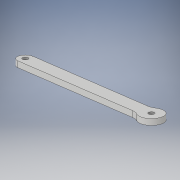
# Autodesk Inventor part: 連接1
Saved by Autodesk Inventor 2017 (Build 210142000, 142)
## iProperties
Part Number: 連接1
Material: 一般
Document SubType Name: Modeling
Designer: User
Density: 1 g/cm^3
Appearance: 預設
Author: User
Autodesk Inventor part; units mm, degrees
ref_plane "YZ Plane" through (0, 0, 0) normal (1, 0, 0) x (0, 1, 0)
ref_plane "XZ Plane" through (0, 0, 0) normal (0, 1, 0) x (-1, 0, 0)
ref_plane "XY Plane" through (0, 0, 0) normal (0, 0, 1) x (1, 0, 0)
sketch "草圖1" plane through (0, 0, 0) normal (0, 1, 0) x (-1, 0, 0)
  circle A0 centre (0, 0) radius 1.5
  circle A1 centre (0, 0) radius 4
  line L0 (0, 0) -> (-80, 0)
  circle A2 centre (-80, 0) radius 1.5
  arc A3 (-76.9095, 5.1429) -> (-76.9095, -5.1429) centre (-80, 0) ccw
  line L1 (0, 4) -> (-72.7889, 4)
  line L2 (0, -4) -> (-72.7889, -4)
  arc A4 (-76.9095, 5.1429) -> (-72.7889, 4) centre (-72.7889, 12) ccw
  arc A5 (-72.7889, -4) -> (-76.9095, -5.1429) centre (-72.7889, -12) ccw
  point P0 (-75.5279, 4)
  point P1 (-75.5279, -4)
  dimension "d0" = 3
  dimension "d1" = 8
  dimension "d2" = 80
  dimension "d3" = 3
  dimension "d4" = 12
  dimension "d5" = 8
  constraints: 10 point on circle, 6 centre point, 6 end point, 4 coincident, 4 tangent, 2 horizontal, 2 point on line, 1 equal radius, 1 parallel
  measures "d0" diameter of A0
  measures "d1" diameter of A1
  measures "d2" distance of L0.start L0.end
  measures "d3" diameter of A2
  measures "d4" diameter of A3
  measures "d5" radius of A4
extrude "擠出1" add sketch "草圖1" along normal mid plane 3
